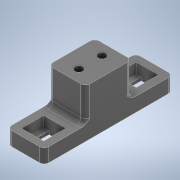
# Autodesk Inventor part: PotHolder
Saved by Autodesk Inventor 2022 (Build 260153000, 153)
## iProperties
Created: 2021-11-22
Part Number: PotHolder
Material: Genérico
Document SubType Name: Modeling
Designer: JK
Density: 1 g/cm^3
Appearance: Suave - Negro
Author: JK
Autodesk Inventor part; units mm, degrees
ref_plane "YZ Plane" through (0, 0, 0) normal (1, 0, 0) x (0, 1, 0)
ref_plane "XZ Plane" through (0, 0, 0) normal (0, 1, 0) x (-1, 0, 0)
ref_plane "XY Plane" through (0, 0, 0) normal (0, 0, 1) x (1, 0, 0)
sketch "Boceto7" plane through (0, 0, 0) normal (0, 1, 0) x (-1, 0, 0)
  line L0 (-8, 12.2) -> (8, 12.2)
  line L1 (8, 12.2) -> (8, -12.2)
  line L2 (8, -12.2) -> (-8, -12.2)
  line L3 (-8, -12.2) -> (-8, 12.2)
  line L4 (-8, 12.2) -> (8, -12.2) construction
  line L5 (8, 12.2) -> (-8, -12.2) construction
  line L6 (8, 12.2) -> (-8, 12.2)
  line L7 (-8, 12.2) -> (-8, 27.8)
  line L8 (-8, 27.8) -> (8, 27.8)
  line L9 (8, 27.8) -> (8, 12.2)
  line L10 (8, -12.2) -> (-8, -12.2)
  line L11 (-8, -12.2) -> (-8, -27.8)
  line L12 (-8, -27.8) -> (8, -27.8)
  line L13 (8, -27.8) -> (8, -12.2)
  line L14 (4.8, 24.8) -> (-4.8, 24.8)
  line L15 (-4.8, 24.8) -> (-4.8, 15.2)
  line L16 (-4.8, 15.2) -> (4.8, 15.2)
  line L17 (4.8, 15.2) -> (4.8, 24.8)
  line L18 (4.8, -15.2) -> (-4.8, -15.2)
  line L19 (-4.8, -15.2) -> (-4.8, -24.8)
  line L20 (-4.8, -24.8) -> (4.8, -24.8)
  line L21 (4.8, -24.8) -> (4.8, -15.2)
  line L22 (-4.8, 24.8) -> (4.8, 24.8)
  line L23 (4.8, 24.8) -> (4.8, 15.2)
  line L24 (4.8, 15.2) -> (-4.8, 15.2)
  line L25 (-4.8, 15.2) -> (-4.8, 24.8)
  line L26 (-4.8, 24.8) -> (4.8, 15.2) construction
  line L27 (4.8, 24.8) -> (-4.8, 15.2) construction
  line L28 (-4.8, -15.2) -> (4.8, -15.2)
  line L29 (4.8, -15.2) -> (4.8, -24.8)
  line L30 (4.8, -24.8) -> (-4.8, -24.8)
  line L31 (-4.8, -24.8) -> (-4.8, -15.2)
  line L32 (-4.8, -15.2) -> (4.8, -24.8) construction
  line L33 (4.8, -15.2) -> (-4.8, -24.8) construction
  point P0 (0, 0)
  point P1 (-8, 12.2)
  point P2 (0, 20)
  point P3 (0, -20)
  point P4 (0, -20)
  point P5 (0, 0)
  dimension "d23" = 9.6
  dimension "d24" = 9.6
  dimension "d26" = 3
  dimension "d28" = 3
  dimension "d30" = 3
  dimension "d31" = 3
  dimension "d43" = 40
  dimension "d48" = 16
  constraints: 68 end point, 14 parallel, 8 midpoint, 7 horizontal, 7 perpendicular, 6 collinear, 2 equal length, 1 point on line, 1 vertical alignment
  measures "d23" distance of L16.end L14.start
  measures "d24" distance of L15.end L16.end
  measures "d26" distance between parallel lines of L14 L8
  measures "d28" distance between parallel lines of L0 L16
  measures "d30" distance between parallel lines of L12 L20
  measures "d31" distance between parallel lines of L2 L18
  measures "d43" distance of point (0, -20) point (0, 20)
  measures "d48" distance between parallel lines of L7 L9
extrude "Extrusión4" add sketch "Boceto7" along normal blind 6
sketch "Boceto8" plane through (0, 6, 0) normal (0, 1, 0) x (1, 0, 0)
  circle A0 centre (0, -4.8061) radius 1.7
  circle A1 centre (0, 5.1939) radius 1.7
  point P0 (0, 0.1939)
  dimension "d35" = 3.4
  dimension "d49" = 5
  dimension "d50" = 5
  constraints: 2 centre point, 2 vertical alignment, 1 equal radius
  measures "d35" diameter of A0
  measures "d49" distance of A0.centre point (0, 0.194)
  measures "d50" distance of point (0, 0.194) A1.centre
extrude "Extrusión5" cut sketch "Boceto8" against normal through all
fillet "Empalme3" radius 2 4 edges at (-8, 3, 27.8) (8, 3, 27.8) (-8, 3, -27.8) (8, 3, -27.8)
sketch "Boceto9" plane through (0, 6, 0) normal (0, 1, 0) x (1, 0, 0)
  line L0 (-8, 25.8) -> (-8, -25.8) projected
  line L1 (8, -10) -> (-8, -10)
  line L2 (-8, -10) -> (-8, 10)
  line L3 (-8, 10) -> (8, 10)
  line L4 (8, 10) -> (8, -10)
  line L5 (8, -10) -> (-8, 10) construction
  line L6 (-8, -10) -> (8, 10) construction
  arc A0 (8, 25.8) -> (6, 27.8) centre (6, 25.8) ccw projected
  line L7 (6, 27.8) -> (-6, 27.8) projected
  arc A1 (-6, 27.8) -> (-8, 25.8) centre (-6, 25.8) ccw projected
  line L8 (-8, 25.8) -> (-8, -25.8) projected
  arc A2 (-8, -25.8) -> (-6, -27.8) centre (-6, -25.8) ccw projected
  line L9 (-6, -27.8) -> (6, -27.8) projected
  arc A3 (6, -27.8) -> (8, -25.8) centre (6, -25.8) ccw projected
  line L10 (8, -25.8) -> (8, 25.8) projected
  circle A4 centre (0, -4.8061) radius 1.7 projected
  line L11 (-4.8, -24.8) -> (-4.8, -15.2) projected
  line L12 (-4.8, -15.2) -> (4.8, -15.2) projected
  line L13 (4.8, -15.2) -> (4.8, -24.8) projected
  line L14 (4.8, -24.8) -> (-4.8, -24.8) projected
  line L15 (-4.8, 15.2) -> (-4.8, 24.8) projected
  line L16 (-4.8, 24.8) -> (4.8, 24.8) projected
  line L17 (4.8, 24.8) -> (4.8, 15.2) projected
  line L18 (4.8, 15.2) -> (-4.8, 15.2) projected
  circle A5 centre (0, 5.1939) radius 1.7 projected
  point P0 (0, 0)
  dimension "d44" = 20
  constraints: 12 end point, 2 midpoint, 2 parallel, 1 horizontal, 1 perpendicular, 1 point on line
  measures "d44" distance between parallel lines of L3 L1
extrude "Extrusión6" add sketch "Boceto9" along normal blind 14.6 contours L3 L4 L1 L0
fillet "Empalme4" radius 2 6 edges at (8, 13.3, 10) (8, 13.3, -10) (-8, 13.3, -10) (-8, 13.3, 10) (0, 6, -10) (0, 6, 10)
sketch "Boceto10" plane through (0, 0, 0) normal (0, -1, 0) x (1, 0, 0)
  circle A0 centre (0, 4.8061) radius 1.7 projected
  circle A1 centre (0, -5.1939) radius 1.7 projected
  arc A2 (6, -27.8) -> (8, -25.8) centre (6, -25.8) ccw projected
  line L0 (8, 25.8) -> (8, -25.8) projected
  arc A3 (8, 25.8) -> (6, 27.8) centre (6, 25.8) ccw projected
  line L1 (-6, 27.8) -> (6, 27.8) projected
  arc A4 (-6, 27.8) -> (-8, 25.8) centre (-6, 25.8) ccw projected
  line L2 (-8, -25.8) -> (-8, 25.8) projected
  arc A5 (-8, -25.8) -> (-6, -27.8) centre (-6, -25.8) ccw projected
  line L3 (6, -27.8) -> (-6, -27.8) projected
  line L4 (-4.8, 24.8) -> (-4.8, 15.2) projected
  line L5 (4.8, 24.8) -> (-4.8, 24.8) projected
  line L6 (4.8, 15.2) -> (4.8, 24.8) projected
  line L7 (-4.8, 15.2) -> (4.8, 15.2) projected
  line L8 (-4.8, -15.2) -> (-4.8, -24.8) projected
  line L9 (4.8, -15.2) -> (-4.8, -15.2) projected
  line L10 (4.8, -24.8) -> (4.8, -15.2) projected
  line L11 (-4.8, -24.8) -> (4.8, -24.8) projected
  line L12 (-4.8, 15.2) -> (4.8, 15.2) projected
  line L13 (-2.4608, 24.8) -> (2.8, 24.8)
  line L14 (2.8, 24.8) -> (2.8, 15.2)
  line L15 (2.8, 15.2) -> (-2.4608, 15.2)
  line L16 (-2.4608, 15.2) -> (-2.4608, 24.8)
  line L17 (-2.4608, 24.8) -> (2.8, 15.2) construction
  line L18 (2.8, 24.8) -> (-2.4608, 15.2) construction
  line L19 (-4.8, -24.8) -> (4.8, -24.8) projected
  line L20 (-2.6635, -15.2) -> (2.8, -15.2)
  line L21 (2.8, -15.2) -> (2.8, -24.8)
  line L22 (2.8, -24.8) -> (-2.6635, -24.8)
  line L23 (-2.6635, -24.8) -> (-2.6635, -15.2)
  line L24 (-2.6635, -15.2) -> (2.8, -24.8) construction
  line L25 (2.8, -15.2) -> (-2.6635, -24.8) construction
  point P0 (0, 0)
  point P1 (0.1696, 20)
  point P2 (0.0682, -20)
  point P3 (2.8, -15.2)
  point P4 (2.8, 24.8)
  dimension "d51" = 2
  constraints: 24 end point, 4 midpoint, 4 parallel, 2 horizontal, 2 perpendicular, 2 point on line, 1 collinear
  measures "d51" distance between parallel lines of L6 L14
extrude "Extrusión7" add sketch "Boceto10" against normal blind 1.4 contours L5 L16 L7 L4 | L5 L6 L7 L14 | L9 L23 L11 L8 | L9 L10 L11 L21
